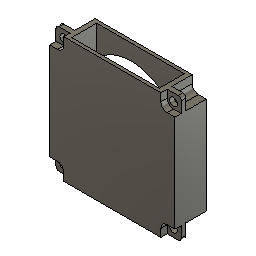
zerofilter_2021-12-16 (Autodesk Fusion 360 archive; units mm, degrees)
design "4010_blower_fan"
Autodesk Fusion 360 part; units mm, degrees
sketch "Sketch1" plane through (0, 0, 0) normal (0, 0, 1) x (1, 0, 0)
  line L0 (0, 0) -> (20, 0)
  line L1 (20, 0) -> (20, 40)
  line L2 (20, 40) -> (0, 40)
  line L3 (0, 40) -> (0, 0)
  line L4 (0, 0) -> (-20, 0)
  line L5 (-20, 0) -> (-20, 40)
  line L6 (-20, 40) -> (0, 40)
  line L7 (0, 40) -> (0, 0)
  circle A0 centre (-3, 20) radius 15
  circle A1 centre (17.5, 37.5) radius 2
  circle A2 centre (-17.5, 37.5) radius 2
  circle A3 centre (-17.5, 2.5) radius 2
  circle A4 centre (17.5, 2.5) radius 2
  line L8 (17.5, 37.5) -> (17.5, 2.5) construction
  line L9 (17.5, 2.5) -> (-17.5, 2.5) construction
  line L10 (-17.5, 37.5) -> (17.5, 37.5) construction
  circle A5 centre (17.5, 37.5) radius 1.25
  circle A6 centre (-17.5, 37.5) radius 1.25
  circle A7 centre (-17.5, 2.5) radius 1.25
  circle A8 centre (17.5, 2.5) radius 1.25
  line L11 (15.5, 37.5) -> (15.5, 40)
  line L12 (17.5, 35.5) -> (20, 35.5)
  line L13 (17.5, 4.5) -> (20, 4.5)
  line L14 (15.5, 2.5) -> (15.5, 0)
  line L15 (-15.5, 2.5) -> (-15.5, 0)
  line L16 (-17.5, 4.5) -> (-20, 4.5)
  line L17 (-17.5, 35.5) -> (-20, 35.5)
  line L18 (-15.5, 37.5) -> (-15.5, 40)
  dimension "d1" = 40
  dimension "d2" = 40
  dimension "d5" = 30
  dimension "d14" = 17.5
  dimension "d16" = 2.5
  dimension "d17" = 2.5
  dimension "d18" = 2.5
  dimension "d19" = 4
  dimension "d29" = 20
  dimension "d30" = 17
  constraint horizontal L0
  constraint vertical L1
  constraint horizontal L2
  constraint vertical L3
  constraint coincident L0.start L3.end
  constraint horizontal L4
  constraint vertical L5
  constraint horizontal L6
  constraint vertical L7
  constraint collinear L2 L6
  constraint equal L0 L4
  constraint coincident A1.centre L8.start
  constraint coincident A4.centre L8.end
  constraint coincident A3.centre L9.end
  constraint coincident A2.centre L10.start
  constraint horizontal L10
  constraint horizontal L9
  constraint vertical L8
  constraint equal L8 L10
  constraint equal L9 L10
  constraint equal A2 A3
  constraint equal A1 A4
  constraint equal A1 A2
  constraint concentric A1 A5
  constraint concentric A2 A6
  constraint concentric A4 A8
  constraint equal A6 A8
  constraint equal A6 A7
  constraint equal A5 A7
  constraint coincident A1 L11.start
  constraint coincident L10 L11.start
  constraint coincident L2 L11.end
  constraint tangent A1 L11
  constraint coincident A1 L12.start
  constraint coincident L8 L12.start
  constraint coincident L1 L12.end
  constraint tangent A1 L12
  constraint coincident A4 L13.start
  constraint coincident L8 L13.start
  constraint coincident L1 L13.end
  constraint tangent A4 L13
  constraint coincident A4 L14.start
  constraint coincident L9 L14.start
  constraint coincident L0 L14.end
  constraint tangent A4 L14
  constraint coincident A3 L15.start
  constraint coincident L9 L15.start
  constraint coincident L4 L15.end
  constraint tangent A3 L15
  constraint coincident A3 L16.start
  constraint coincident L5 L16.end
  constraint tangent A3 L16
  constraint perpendicular L5 L16
  constraint coincident A2 L17.start
  constraint coincident L5 L17.end
  constraint tangent A2 L17
  constraint perpendicular L5 L17
  constraint coincident L10 L18.start
  constraint coincident A2 L18.start
  constraint coincident L6 L18.end
  constraint tangent A2 L18
  measures "d1" distance of L0.end L1.end
  measures "d2" distance of L1 L5
  measures "d5" diameter of A0
  measures "d14" distance of L7 L8
  measures "d16" distance of L2 L10
  measures "d17" distance of L0 L9
  measures "d18" diameter of A5
  measures "d19" diameter of A1
  measures "d29" distance of L4 A0.centre
  measures "d30" distance of L5 A0.centre
extrude "Extrude1" add sketch "Sketch1" along normal blind 10 contours L0 L1 L2 L3 L7 A0 A1 A4 L11 L12 L13 L14 | L3 L4 L5 L6 L7 A0 A2 A3 L15 L16 L17 L18 | L0 L1 A4 L13 L14 | L3 L7 A0 | L3 L7 A0 | L4 L5 A3 L15 L16 | A4 | A3 | L1 L2 A1 L11 L12 | L5 L6 A2 L17 L18 | A1 | A2 | A5 | A6 | A7 | A8
extrude "Extrude2" cut sketch "Sketch1" along normal blind 9 contours L3 L7 A0 | L3 L7 A0
sketch "Sketch2" plane through (0, 40, 0) normal (0, 1, 0) x (-1, 0, 0)
  line L0 (-20, 0) -> (20, 0)
  line L1 (20, 0) -> (20, 10)
  line L2 (20, 10) -> (-20, 10)
  line L3 (-20, 10) -> (-20, 0)
  line L4 (-14, 1) -> (14, 1)
  line L5 (14, 1) -> (14, 9)
  line L6 (14, 9) -> (-14, 9)
  line L7 (-14, 9) -> (-14, 1)
  line L8 (-14, 1) -> (14, 9) construction
  line L9 (14, 1) -> (-14, 9) construction
  line L10 (0, 5) -> (0, 0) construction
  line L11 (0, 5) -> (-20, 5) construction
  point P0 (0, 5)
  dimension "d9" = 28
  dimension "d10" = 8
  constraint horizontal L4
  constraint perpendicular L4 L5
  constraint parallel L4 L6
  constraint parallel L5 L7
  constraint coincident L8 P0
  constraint coincident L9 P0
  constraint coincident P0 L10.start
  constraint coincident L10.end origin
  constraint midpoint L3 L11.end
  constraint vertical L10
  constraint horizontal L11
  measures "d9" distance of L4.start L4.end
  measures "d10" distance of L4 L6
extrude "Extrude3" cut sketch "Sketch2" against normal blind 17 contours L4 L5 L6 L7
extrude "Extrude4" cut sketch "Sketch1" along normal blind 6.5 contours L0 L1 A4 L13 L14 | L4 L5 A3 L15 L16 | A4 | A3 | L1 L2 A1 L11 L12 | L5 L6 A2 L17 L18 | A1 | A2 | A5 | A6 | A7 | A8
extrude "Extrude5" cut sketch "Sketch1" along normal blind 44 contours A5 | A6 | A7 | A8
sketch "Sketch3" plane through (0, 0, 10) normal (0, 0, 1) x (1, 0, 0)
  circle A0 centre (-17.5, 37.5) radius 1.25
  circle A1 centre (-17.5, 2.5) radius 1.25
  circle A2 centre (17.5, 37.5) radius 1.25
  circle A3 centre (17.5, 2.5) radius 1.25
  line L0 (-20, 0) -> (20, 0)
  line L1 (20, 0) -> (20, 40)
  line L2 (20, 40) -> (-20, 40)
  line L3 (-20, 40) -> (-20, 0)
  circle A4 centre (-17.5, 37.5) radius 1.25
  arc A5 (-17.5, 35.5) -> (-15.5, 37.5) centre (-17.5, 37.5) ccw
  line L4 (-17.5, 35.5) -> (-20, 35.5)
  line L5 (-20, 35.5) -> (-20, 40)
  line L6 (-20, 40) -> (-15.5, 40)
  line L7 (-15.5, 40) -> (-15.5, 37.5)
  circle A6 centre (17.5, 37.5) radius 1.25
  arc A7 (15.5, 37.5) -> (17.5, 35.5) centre (17.5, 37.5) ccw
  line L8 (15.5, 37.5) -> (15.5, 40)
  line L9 (15.5, 40) -> (20, 40)
  line L10 (20, 40) -> (20, 35.5)
  line L11 (20, 35.5) -> (17.5, 35.5)
  circle A8 centre (-17.5, 2.5) radius 1.25
  arc A9 (-15.5, 2.5) -> (-17.5, 4.5) centre (-17.5, 2.5) ccw
  line L12 (-15.5, 2.5) -> (-15.5, 0)
  line L13 (-15.5, 0) -> (-20, 0)
  line L14 (-20, 0) -> (-20, 4.5)
  line L15 (-20, 4.5) -> (-17.5, 4.5)
  circle A10 centre (17.5, 2.5) radius 1.25
  arc A11 (17.5, 4.5) -> (15.5, 2.5) centre (17.5, 2.5) ccw
  line L16 (17.5, 4.5) -> (20, 4.5)
  line L17 (20, 4.5) -> (20, 0)
  line L18 (20, 0) -> (15.5, 0)
  line L19 (15.5, 0) -> (15.5, 2.5)
extrude "Extrude6" cut sketch "Sketch3" against normal blind 2 contours L0 L3 A9 L12 L13 L14 L15 | L0 L1 A11 L16 L17 L18 L19 | L2 L3 A5 L4 L5 L6 L7 | L1 L2 A7 L8 L9 L10 L11
fillet "Fillet1" radius 1 4 edges at (-20, 0, 7.25) (-20, 40, 7.25) (20, 0, 7.25) (20, 40, 7.25)
equation "d11 = -34.00 mm / 2"
